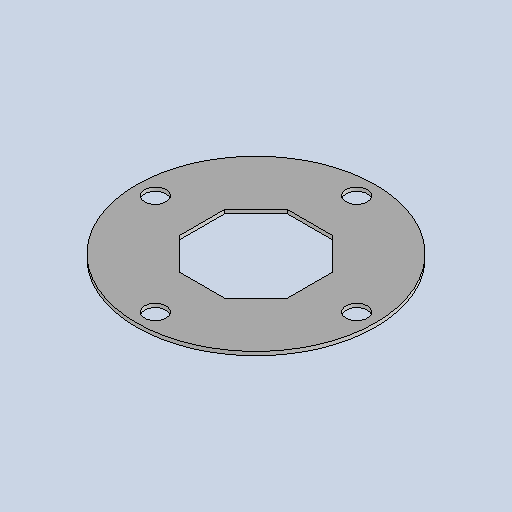
# Autodesk Inventor part: PNS 1792  funnel FLANGE 1200 50-90_1000x90
Saved by Autodesk Inventor 2025.1 (Build 291241020, 241B)
## iProperties
Created: 2025-06-24
Part Number: PNS 1792  funnel FLANGE 1200 50-90_1000x90
Material: Stainless Steel
Description: DIE16(5)|\ 90°|corrY -___°|X_____|bom___
Document SubType Name: Sheet Metal
Designer: user
Mass: 511.175 g
Surface Area: 458.858 cm^2
Volume: 63.8969 cm^3
Density: 8 g/cm^3
Flat Pattern Width: 19 cm
Flat Pattern Length: 19 cm
Flat Pattern Area: 361 cm^2
Sheet Metal Rule: Default
Sheet Metal Width: 190.000 mm
Sheet Metal Length: 190.000 mm
Sheet Metal Area: 36100.000 mm^2
Appearance: Default
Author: user
Autodesk Inventor part; units mm, degrees
ref_plane "YZ Plane" through (0, 0, 0) normal (1, 0, 0) x (0, 1, 0)
ref_plane "XZ Plane" through (0, 0, 0) normal (0, 1, 0) x (-1, 0, 0)
ref_plane "XY Plane" through (0, 0, 0) normal (0, 0, 1) x (1, 0, 0)
sketch "Sketch1" plane through (0, 0, 0) normal (0, 0, 1) x (1, 0, 0)
  circle A0 centre (0, 0) radius 95
  line L0 (43, 43) -> (-43, 43)
  line L1 (-43, 43) -> (-43, -43)
  line L2 (-43, -43) -> (43, -43)
  line L3 (43, -43) -> (43, 43)
  line L4 (43, 43) -> (-43, -43) construction
  line L5 (-43, 43) -> (43, -43) construction
  dimension "d157" = 190
  dimension "d158" = 86
  dimension "d159" = 86
  measures "d157" diameter of A0
  measures "d158" distance of L2.end L1.end
  measures "d159" distance of L1.end L0.end
extrude "Plate5" add sketch "Sketch1" along normal blind 3
sketch "Sketch7" plane through (0, 0, 0) normal (0, 0, -1) x (-1, 0, 0)
  circle A0 centre (0, 80) radius 8.5
  point P0 (0, 0)
  dimension "d160" = 17
  dimension "d161" = 80
  constraints: 1 centre point, 1 vertical alignment
  measures "d160" diameter of A0
  measures "d161" distance of point (0, 0) A0.centre
extrude "Cut1" cut sketch "Sketch7" against normal blind 3
pattern_circular "Circular Pattern1" count 4 over 360 about axis through (0, 0, -10) along (0, 0, 1) of "Cut1"
chamfer "Corner Chamfer2" distance 25 angle 45 4 edges at (-43, -43, 1.5) (43, -43, 1.5) (-43, 43, 1.5) (43, 43, 1.5)
body "Solid3"
